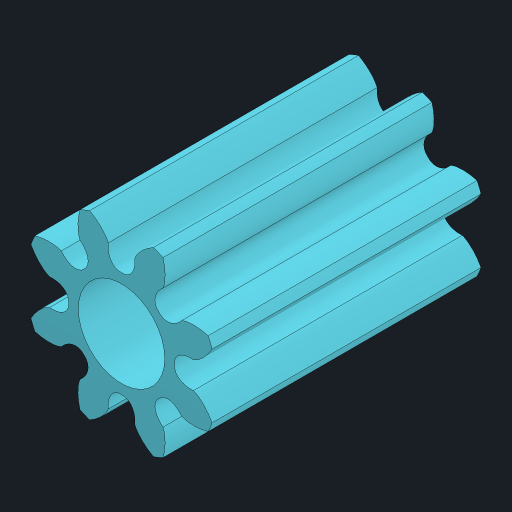
# Autodesk Inventor part: Idler Gear
Saved by Autodesk Inventor 2023.2 (Build 272271030, 271C)
## iProperties
Created: 2024-02-19
Part Number: Idler Gear
Material: Generic
Document SubType Name: Modeling
Designer: robpl
Density: 1 g/cm^3
Appearance: Cadet Blue
Author: robpl
Autodesk Inventor part; units mm, degrees
ref_plane "YZ Plane" through (0, 0, 0) normal (1, 0, 0) x (0, 1, 0)
ref_plane "XZ Plane" through (0, 0, 0) normal (0, 1, 0) x (-1, 0, 0)
ref_plane "XY Plane" through (0, 0, 0) normal (0, 0, 1) x (1, 0, 0)
sketch "Sketch1" plane through (0, 0, 0) normal (0, 0, 1) x (1, 0, 0)
  spline S0 degree 3 poles (-1.6607, 4.7162) (-1.6104, 4.687) (-1.5097, 4.6286) (-1.3654, 4.5302) (-1.2269, 4.4238) (-1.0958, 4.3084) (-0.9735, 4.1837) (-0.8806, 4.0715) (-0.8132, 3.9766) (-0.767, 3.9026) (-0.7251, 3.8259) (-0.7034, 3.7719) (-0.6925, 3.7449) knots 0 0 0 0 0.125007 0.250017 0.375024 0.500027 0.625023 0.750007 0.812514 0.875018 0.937517 1 1 1 1
  spline S1 degree 3 poles (-0.6925, 3.7449) (-0.6949, 3.716) (-0.6996, 3.6582) (-0.6997, 3.5711) (-0.6945, 3.4842) (-0.6848, 3.3977) (-0.6675, 3.3124) (-0.6447, 3.2283) (-0.6133, 3.1471) (-0.5749, 3.0689) (-0.528, 2.9954) (-0.4724, 2.9283) (-0.4084, 2.869) (-0.3363, 2.8198) (-0.2576, 2.782) (-0.1877, 2.7619) (-0.1305, 2.7522) (-0.0725, 2.7487) (0, 2.7508) (0.0725, 2.7487) (0.1305, 2.7522) (0.1877, 2.7619) (0.2576, 2.782) (0.3363, 2.8198) (0.4084, 2.869) (0.4724, 2.9283) (0.528, 2.9954) (0.5749, 3.0689) (0.6133, 3.1471) (0.6447, 3.2283) (0.6675, 3.3124) (0.6848, 3.3977) (0.6945, 3.4842) (0.6997, 3.5711) (0.6996, 3.6582) (0.6949, 3.716) (0.6925, 3.7449) knots 0 0 0 0 0.031256 0.062517 0.093774 0.12503 0.156284 0.187541 0.218792 0.250037 0.281288 0.312538 0.343783 0.375021 0.406258 0.437484 0.453123 0.468742 0.5 0.531258 0.546877 0.562516 0.593742 0.624979 0.656217 0.687462 0.718712 0.749963 0.781208 0.812459 0.843716 0.87497 0.906226 0.937483 0.968744 1 1 1 1
  spline S2 degree 3 poles (0.6925, 3.7449) (0.7034, 3.7719) (0.7251, 3.8259) (0.767, 3.9026) (0.8132, 3.9766) (0.8806, 4.0715) (0.9735, 4.1837) (1.0958, 4.3084) (1.2269, 4.4238) (1.3654, 4.5302) (1.5097, 4.6286) (1.6104, 4.687) (1.6607, 4.7162) knots 0 0 0 0 0.062483 0.124982 0.187486 0.249993 0.374977 0.499973 0.624976 0.749983 0.874993 1 1 1 1
  circle A0 centre (0, 0) radius 2.75 construction
  circle A1 centre (0, 0) radius 3.7588 construction
  circle A2 centre (0, 0) radius 4 construction
  circle A3 centre (0, 0) radius 5
  point P0 (-1.5108, 4.6268)
  point P1 (-1.3663, 4.5289)
  point P2 (-1.2281, 4.4223)
  point P3 (-1.0973, 4.3069)
  point P4 (-0.9753, 4.182)
  point P5 (-0.8644, 4.0474)
  point P6 (-0.814, 3.9761)
  point P7 (-0.7677, 3.9021)
  point P8 (-0.7266, 3.8252)
  point P9 (-0.6984, 3.6581)
  point P10 (-0.6988, 3.5711)
  point P11 (-0.6937, 3.4843)
  point P12 (-0.6835, 3.3979)
  point P13 (-0.6666, 3.3126)
  point P14 (-0.6432, 3.2288)
  point P15 (-0.6121, 3.1476)
  point P16 (-0.5735, 3.0697)
  point P17 (-0.5266, 2.9965)
  point P18 (-0.471, 2.9296)
  point P19 (-0.407, 2.8707)
  point P20 (-0.3352, 2.8217)
  point P21 (-0.2567, 2.7843)
  point P22 (-0.1733, 2.76)
  point P23 (-0.1304, 2.753)
  point P24 (-0.087, 2.75)
  point P25 (0, 2.75)
  point P26 (0.087, 2.75)
  point P27 (0.1304, 2.753)
  point P28 (0.1733, 2.76)
  point P29 (0.2567, 2.7843)
  point P30 (0.3352, 2.8217)
  point P31 (0.407, 2.8707)
  point P32 (0.471, 2.9296)
  point P33 (0.5266, 2.9965)
  point P34 (0.5735, 3.0697)
  point P35 (0.6121, 3.1476)
  point P36 (0.6432, 3.2288)
  point P37 (0.6666, 3.3126)
  point P38 (0.6835, 3.3979)
  point P39 (0.6937, 3.4843)
  point P40 (0.6988, 3.5711)
  point P41 (0.6984, 3.6581)
  point P42 (0.7266, 3.8252)
  point P43 (0.7677, 3.9021)
  point P44 (0.814, 3.9761)
  point P45 (0.8644, 4.0474)
  point P46 (0.9753, 4.182)
  point P47 (1.0973, 4.3069)
  point P48 (1.2281, 4.4223)
  point P49 (1.3663, 4.5289)
  point P50 (1.5108, 4.6268)
  constraints: 4 centre point, 2 point on circle, 117 other
extrude "Extrusion1" add sketch "Sketch1" against normal blind 14
extrude "Extrusion2" cut sketch "Sketch1" against normal through all contours A3 S2 S1 S0 picked at (0.1954, 4.3023)
pattern_circular "Circular Pattern1" count 8 over 360 about axis through (0, 0, 0) along (0, 0, -1) of "Extrusion2"
sketch "Sketch2" plane through (0, 0, 0) normal (0, 0, 1) x (1, 0, 0)
  point P0 (0, 0)
  point P1 (0, 0)
  constraints: 1 coincident
hole "Hole1" at (0, 0, 0) direction (0, 0, -1) diameter 2.5 end through all counterbore diameter 4.5 counterbore depth 5.8
equation "\"Module\" = 1"
equation "\"PressureAngle\" = 20deg"
equation "\"UnitProfileClearance\" = 0.25"
equation "\"UnitRoundRadius\" = 0.35"
equation "\"RootDiameter\" = 5.5"
equation "\"BaseDiameter\" = 7.51754"
equation "\"PitchDiameter\" = 8"
equation "\"HelixAngle\" = 0"
equation "\"UnitCorrection\" = 0"
equation "\"UnitAddendumModification\" = 0"
equation "\"CircularPitch\" = 3.141593"
equation "\"UnitBacklashShift\" = 0"
equation "\"TotalToolShift\" = 0"
equation "\"IsInternal\" = 0"
body "Solid1"
